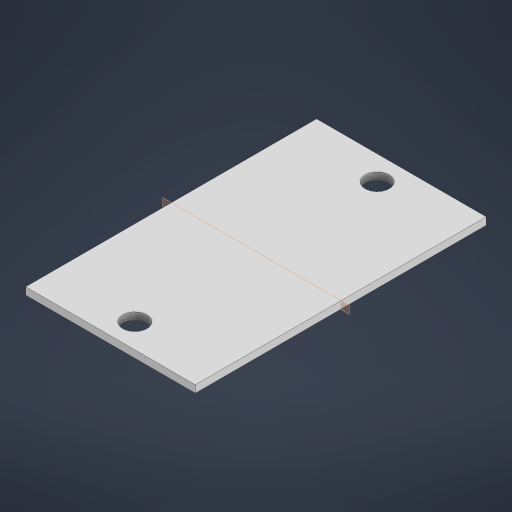
# Autodesk Inventor part: adafruit_TCA9548A_board
Saved by Autodesk Inventor 2024 (Build 280153000, 153)
## iProperties
Created: 2026-03-30
Part Number: adafruit_TCA9548A_board
Material: Generic
Document SubType Name: Modeling
Designer: schar
Density: 1 g/cm^3
Appearance: Default
Author: schar
Autodesk Inventor part; units mm, degrees
ref_plane "YZ Plane" through (0, 0, 0) normal (1, 0, 0) x (0, 1, 0)
ref_plane "XZ Plane" through (0, 0, 0) normal (0, 1, 0) x (-1, 0, 0)
ref_plane "XY Plane" through (0, 0, 0) normal (0, 0, 1) x (1, 0, 0)
sketch "Sketch1" plane through (0, 0, 0) normal (0, 1, 0) x (-1, 0, 0)
  line L0 (8.89, 15.24) -> (-8.89, 15.24)
  line L1 (-8.89, 15.24) -> (-8.89, -15.24)
  line L2 (-8.89, -15.24) -> (8.89, -15.24)
  line L3 (8.89, -15.24) -> (8.89, 15.24)
  line L4 (8.89, 15.24) -> (-8.89, -15.24) construction
  line L5 (-8.89, 15.24) -> (8.89, -15.24) construction
  line L6 (8.89, 0) -> (8.89, -12.7)
  line L7 (8.89, 0) -> (8.89, 12.7)
  line L8 (8.89, 15.24) -> (0, 15.24)
  circle A0 centre (0, 12.7) radius 1.27
  circle A1 centre (0, -12.7) radius 1.27
  point P0 (0, 0)
  dimension "d0" = 17.78
  dimension "d1" = 30.48
  dimension "d2" = 12.7
  dimension "d3" = 12.7
  dimension "d4" = 8.89
  dimension "d5" = 2.54
  dimension "d6" = 2.54
  constraints: 18 end point, 4 midpoint, 2 centre point, 2 coincident, 2 parallel, 1 collinear, 1 horizontal, 1 perpendicular, 1 point on line
  measures "d0" distance of L2.end L1.end
  measures "d1" distance of L1.end L0.end
  measures "d2" distance of L6.start L6.end
  measures "d3" distance of L6.start L7.end
  measures "d4" distance of L0.start L8.end
  measures "d5" diameter of A0
  measures "d6" diameter of A1
extrude "Extrusion1" add sketch "Sketch1" along normal blind 0.762
ref_plane "Work Plane1" through (-8.89, 0, 0) normal (0, 0, 1) x (1, 0, 0)
body "Solid1"
